Santa Body v25 (Autodesk Fusion 360 design; units mm, degrees)
Autodesk Fusion 360 part; units mm, degrees
sketch "Sketch1" plane through (0, 0, 0) normal (0, 1, 0) x (1, 0, 0)
  line L0 (55.0356, 82.2427) -> (55.0356, 73.8917)
  spline S0 degree 3 poles (10.235, 105.7553) (11.1266, 105.7379) (11.5873, 104.8858) (11.5794, 104.5647) knots 0 0 0 0 1 1 1 1
  spline S1 degree 3 poles (55.0356, 82.2427) (55.0356, 83.8658) (53.7211, 85.1817) (52.0987, 85.1817) knots 0 0 0 0 1 1 1 1
  spline S2 degree 3 poles (38.6811, 112.0285) (38.6811, 112.3322) (38.9274, 112.5785) (39.2311, 112.5785) knots 0 0 0 0 1 1 1 1
  spline S3 degree 3 poles (22.9591, 112.0969) (22.9591, 112.4007) (23.2054, 112.6469) (23.5091, 112.6469) knots 0 0 0 0 1 1 1 1
  spline S4 degree 3 poles (18.5903, 27.8928) (18.5903, 29.3352) (19.3689, 30.5045) (21.0261, 30.5045) knots 0 0 0 0 1 1 1 1
  spline S5 degree 3 poles (26.8266, 106.1753) (27.7269, 106.1753) (28.4266, 105.5866) (28.4565, 104.8612) knots 0 0 0 0 1 1 1 1
  spline S6 degree 3 poles (45.7572, 114.0087) (45.481, 114.0087) (45.2572, 114.2326) (45.2572, 114.5087) knots 0 0 0 0 1 1 1 1
  spline S7 degree 3 poles (10.235, 114.5284) (8.6125, 114.5284) (7.297, 113.2125) (7.297, 111.5894) knots 0 0 0 0 1 1 1 1
  line L1 (39.2311, 111.5335) -> (39.2311, 112.5235)
  line L2 (21.4641, 112.0969) -> (20.4741, 112.0969)
  spline S8 degree 3 poles (14.5168, 97.0703) (12.8944, 97.0703) (11.5794, 95.7544) (11.5794, 94.1313) knots 0 0 0 0 1 1 1 1
  spline S9 degree 3 poles (52.0987, 42.6031) (51.0209, 42.5992) (50.737, 43.4395) (50.7482, 43.786) knots 0 0 0 0 1 1 1 1
  line L3 (33.1192, 46.765) -> (30.3886, 46.7831)
  line L4 (29.7315, 25.7971) -> (29.7315, 27.8928)
  line L5 (45.7572, 114.9587) -> (45.7572, 114.0587)
  spline S10 degree 3 poles (11.5794, 43.7193) (11.5828, 43.2312) (11.1144, 42.5873) (10.235, 42.6031) knots 0 0 0 0 1 1 1 1
  spline S11 degree 3 poles (14.8657, 84.9034) (14.1399, 84.9034) (13.362, 85.633) (13.362, 86.5333) knots 0 0 0 0 1 1 1 1
  line L6 (47.8108, 120.2947) -> (14.5168, 120.2947)
  line L7 (39.2311, 112.5235) -> (39.2311, 111.5335)
  line L8 (13.362, 87.7791) -> (13.362, 86.5333)
  line L9 (11.5794, 117.3562) -> (11.5794, 115.708)
  spline S12 degree 3 poles (47.8108, 100.5358) (49.4323, 100.5897) (50.7482, 101.8518) (50.7482, 103.4749) knots 0 0 0 0 1 1 1 1
  spline S13 degree 3 poles (20.5642, 104.8612) (20.5642, 105.587) (21.2944, 106.1753) (22.1947, 106.1753) knots 0 0 0 0 1 1 1 1
  line L10 (27.1821, 15.6906) -> (27.1821, 15.8565)
  spline S14 degree 3 poles (39.2311, 112.5785) (39.5349, 112.5785) (39.7811, 112.3322) (39.7811, 112.0285) knots 0 0 0 0 1 1 1 1
  spline S15 degree 3 poles (21.5191, 112.0969) (21.5191, 111.7932) (21.2729, 111.5469) (20.9691, 111.5469) knots 0 0 0 0 1 1 1 1
  line L11 (46.2072, 114.5087) -> (45.7572, 114.5087)
  spline S16 degree 3 poles (34.2572, 114.5087) (34.2572, 114.7849) (34.481, 115.0087) (34.7572, 115.0087) knots 0 0 0 0 1 1 1 1
  line L12 (34.7572, 114.0587) -> (34.7572, 114.9587)
  line L13 (7.297, 73.8917) -> (7.297, 82.2427)
  line L14 (21.0261, 30.5045) -> (27.2951, 30.5045)
  line L15 (34.7572, 114.5087) -> (34.3072, 114.5087)
  line L16 (45.3072, 114.5087) -> (46.2072, 114.5087)
  line L17 (47.8108, 97.0703) -> (31.1635, 97.0703)
  line L18 (11.5794, 94.1313) -> (11.5794, 86.3718)
  line L19 (11.5794, 104.5647) -> (11.5794, 103.4749)
  line L20 (33.0945, 89.2552) -> (33.1192, 46.765)
  line L21 (45.7572, 114.5087) -> (45.3072, 114.5087)
  spline S17 degree 3 poles (34.7572, 114.9587) (35.0057, 114.9587) (35.2072, 114.7573) (35.2072, 114.5087) knots 0 0 0 0 1 1 1 1
  spline S18 degree 3 poles (29.7315, 25.7971) (29.7315, 24.3547) (28.9523, 23.1855) (27.2951, 23.1855) knots 0 0 0 0 1 1 1 1
  spline S19 degree 3 poles (35.3373, 12.025) (36.9598, 12.025) (38.2753, 13.3404) (38.2753, 14.9635) knots 0 0 0 0 1 1 1 1
  line L22 (30.3965, 89.2751) -> (33.0945, 89.2552)
  spline S20 degree 3 poles (20.9691, 111.5469) (20.6654, 111.5469) (20.4191, 111.7932) (20.4191, 112.0969) knots 0 0 0 0 1 1 1 1
  spline S21 degree 3 poles (50.7482, 104.5729) (50.749, 105.0607) (51.0594, 105.7079) (52.0987, 105.7553) knots 0 0 0 0 1 1 1 1
  spline S22 degree 3 poles (39.2311, 111.4785) (38.9274, 111.4785) (38.6811, 111.7247) (38.6811, 112.0285) knots 0 0 0 0 1 1 1 1
  line L23 (24.0041, 112.0969) -> (23.0141, 112.0969)
  spline S23 degree 3 poles (55.0356, 111.5894) (55.0356, 113.2125) (53.7211, 114.5284) (52.0987, 114.5284) knots 0 0 0 0 1 1 1 1
  line L24 (50.7482, 69.7345) -> (50.7482, 43.786)
  spline S24 degree 3 poles (50.7482, 69.7345) (50.7292, 70.4446) (51.1934, 70.9205) (52.0987, 70.9521) knots 0 0 0 0 1 1 1 1
  spline S25 degree 3 poles (52.0987, 105.7553) (53.7211, 105.7553) (55.0356, 107.0707) (55.0356, 108.6938) knots 0 0 0 0 1 1 1 1
  line L25 (11.5794, 86.3718) -> (11.5794, 94.1313)
  line L26 (34.3072, 114.5087) -> (35.2072, 114.5087)
  spline S26 degree 3 poles (45.2572, 114.5087) (45.2572, 114.7849) (45.481, 115.0087) (45.7572, 115.0087) knots 0 0 0 0 1 1 1 1
  spline S27 degree 3 poles (15.2169, 89.409) (15.9427, 89.409) (16.7206, 88.6794) (16.7206, 87.7791) knots 0 0 0 0 1 1 1 1
  line L27 (11.5794, 43.7193) -> (11.5794, 69.7582)
  spline S28 degree 3 poles (52.0987, 70.9521) (53.7202, 71.006) (55.0356, 72.2686) (55.0356, 73.8917) knots 0 0 0 0 1 1 1 1
  line L28 (13.362, 86.5333) -> (13.362, 87.7791)
  line L29 (55.0356, 111.5894) -> (55.0356, 108.6938)
  spline S29 degree 3 poles (7.297, 31.3131) (7.297, 29.69) (8.6125, 28.374) (10.235, 28.374) knots 0 0 0 0 1 1 1 1
  line L30 (0.1406, 0.1406) -> (0.1406, 121.8594)
  line L31 (14.8657, 89.409) -> (15.2169, 89.409)
  spline S30 degree 3 poles (41.7711, 112.5785) (42.0749, 112.5785) (42.3211, 112.3322) (42.3211, 112.0285) knots 0 0 0 0 1 1 1 1
  line L32 (14.5168, 16.4854) -> (22.8385, 16.4854)
  line L33 (18.5903, 27.8928) -> (18.5903, 25.7971)
  line L34 (39.2311, 112.0285) -> (39.7261, 112.0285)
  line L35 (18.5903, 25.7971) -> (18.5903, 27.8928)
  spline S31 degree 3 poles (28.4565, 104.6953) (28.4565, 103.9695) (27.7269, 103.3812) (26.8266, 103.3812) knots 0 0 0 0 1 1 1 1
  line L36 (14.8657, 84.9034) -> (15.2169, 84.9034)
  spline S32 degree 3 poles (41.7711, 111.4785) (41.4674, 111.4785) (41.2211, 111.7247) (41.2211, 112.0285) knots 0 0 0 0 1 1 1 1
  spline S33 degree 3 poles (50.7482, 94.1313) (50.7482, 95.7544) (49.4332, 97.0703) (47.8108, 97.0703) knots 0 0 0 0 1 1 1 1
  spline S34 degree 3 poles (16.7206, 86.5333) (16.7206, 85.633) (15.9423, 84.9332) (15.2169, 84.9034) knots 0 0 0 0 1 1 1 1
  line L37 (30.3886, 46.7831) -> (30.3965, 89.2751)
  line L38 (41.2761, 112.0285) -> (41.7711, 112.0285)
  spline S35 degree 3 poles (35.0744, 15.6906) (35.0744, 14.9648) (34.3442, 14.3765) (33.4439, 14.3765) knots 0 0 0 0 1 1 1 1
  spline S36 degree 3 poles (39.2311, 111.5335) (38.9578, 111.5335) (38.7361, 111.7551) (38.7361, 112.0285) knots 0 0 0 0 1 1 1 1
  spline S37 degree 3 poles (34.7572, 115.0087) (35.0333, 115.0087) (35.2572, 114.7849) (35.2572, 114.5087) knots 0 0 0 0 1 1 1 1
  line L39 (28.4565, 104.6953) -> (28.4565, 104.8612)
  line L40 (33.4439, 14.3765) -> (28.812, 14.3765)
  spline S38 degree 3 poles (10.235, 70.9521) (11.1129, 70.9036) (11.6031, 70.3892) (11.5794, 69.7582) knots 0 0 0 0 1 1 1 1
  line L41 (28.812, 17.1706) -> (33.4439, 17.1706)
  line L42 (11.5794, 115.708) -> (11.5794, 117.3562)
  line L43 (20.9691, 111.6019) -> (20.9691, 112.5919)
  line L44 (0.1406, 121.8594) -> (61.8594, 121.8594)
  line L45 (7.297, 31.3131) -> (7.297, 39.6646)
  line L46 (42.2661, 112.0285) -> (41.2761, 112.0285)
  line L47 (7.297, 39.6646) -> (7.297, 31.3131)
  line L48 (11.5794, 27.2452) -> (11.5794, 19.4245)
  line L49 (35.0744, 15.6906) -> (35.0744, 15.8565)
  spline S39 degree 3 poles (24.0041, 112.0969) (24.0041, 112.3703) (23.7825, 112.5919) (23.5091, 112.5919) knots 0 0 0 0 1 1 1 1
  line L50 (27.2951, 30.5045) -> (21.0261, 30.5045)
  line L51 (27.1821, 15.8565) -> (27.1821, 15.6906)
  spline S40 degree 3 poles (41.2211, 112.0285) (41.2211, 112.3322) (41.4674, 112.5785) (41.7711, 112.5785) knots 0 0 0 0 1 1 1 1
  line L52 (28.4565, 104.8612) -> (28.4565, 104.6953)
  spline S41 degree 3 poles (23.5091, 111.6019) (23.2357, 111.6019) (23.0141, 111.8236) (23.0141, 112.0969) knots 0 0 0 0 1 1 1 1
  line L53 (7.297, 111.5894) -> (7.297, 108.6938)
  spline S42 degree 3 poles (46.2572, 114.5087) (46.2572, 114.2326) (46.0333, 114.0087) (45.7572, 114.0087) knots 0 0 0 0 1 1 1 1
  spline S43 degree 3 poles (47.8108, 16.4854) (49.4323, 16.5393) (50.7482, 17.8014) (50.7482, 19.4245) knots 0 0 0 0 1 1 1 1
  spline S44 degree 3 poles (20.9691, 111.6019) (20.6957, 111.6019) (20.4741, 111.8236) (20.4741, 112.0969) knots 0 0 0 0 1 1 1 1
  spline S45 degree 3 poles (42.2661, 112.0285) (42.2661, 112.3019) (42.0445, 112.5235) (41.7711, 112.5235) knots 0 0 0 0 1 1 1 1
  line L54 (35.0744, 15.8565) -> (35.0744, 15.6906)
  line L55 (50.7482, 19.4245) -> (50.7482, 27.1735)
  line L56 (35.2072, 114.5087) -> (34.7572, 114.5087)
  spline S46 degree 3 poles (24.0591, 112.0969) (24.0591, 111.7932) (23.8129, 111.5469) (23.5091, 111.5469) knots 0 0 0 0 1 1 1 1
  line L57 (22.1947, 103.3812) -> (26.8266, 103.3812)
  line L58 (22.8385, 16.4854) -> (14.5168, 16.4854)
  spline S47 degree 3 poles (45.7572, 114.9587) (46.0057, 114.9587) (46.2072, 114.7573) (46.2072, 114.5087) knots 0 0 0 0 1 1 1 1
  line L59 (26.9903, 12.025) -> (35.3373, 12.025)
  line L60 (27.2951, 23.1855) -> (21.0261, 23.1855)
  line L61 (50.7482, 117.3562) -> (50.7482, 115.7102)
  spline S48 degree 3 poles (50.7482, 27.1735) (50.7463, 28.0057) (51.624, 28.3964) (52.0987, 28.374) knots 0 0 0 0 1 1 1 1
  spline S49 degree 3 poles (27.2951, 30.5045) (28.9523, 30.5045) (29.7315, 29.3352) (29.7315, 27.8928) knots 0 0 0 0 1 1 1 1
  line L62 (50.7482, 43.786) -> (50.7482, 69.7345)
  line L63 (21.0261, 23.1855) -> (27.2951, 23.1855)
  line L64 (50.7482, 103.4749) -> (50.7482, 104.5729)
  spline S50 degree 3 poles (27.1821, 15.8565) (27.1821, 16.5823) (27.9117, 17.1706) (28.812, 17.1706) knots 0 0 0 0 1 1 1 1
  spline S51 degree 3 poles (11.5794, 86.3718) (11.585, 85.8428) (11.1354, 85.1501) (10.235, 85.1817) knots 0 0 0 0 1 1 1 1
  spline S52 degree 3 poles (11.5794, 103.4749) (11.5794, 101.8518) (12.8944, 100.5358) (14.5168, 100.5358) knots 0 0 0 0 1 1 1 1
  line L65 (41.7711, 112.5235) -> (41.7711, 111.5335)
  spline S53 degree 3 poles (38.2753, 14.9635) (38.2769, 16.2773) (39.0062, 16.4966) (39.4957, 16.4854) knots 0 0 0 0 1 1 1 1
  line L66 (20.4741, 112.0969) -> (20.9691, 112.0969)
  spline S54 degree 3 poles (52.0987, 85.1817) (51.0422, 85.1715) (50.7324, 85.8189) (50.7482, 86.3525) knots 0 0 0 0 1 1 1 1
  spline S55 degree 3 poles (50.7482, 117.3562) (50.7482, 118.9793) (49.4332, 120.2947) (47.8108, 120.2947) knots 0 0 0 0 1 1 1 1
  line L67 (23.5091, 111.6019) -> (23.5091, 112.5919)
  line L68 (20.5642, 104.8612) -> (20.5642, 104.6953)
  spline S56 degree 3 poles (10.235, 85.1817) (8.6125, 85.1817) (7.297, 83.8658) (7.297, 82.2427) knots 0 0 0 0 1 1 1 1
  line L69 (47.8108, 100.5358) -> (14.5168, 100.5358)
  spline S57 degree 3 poles (20.9691, 112.6469) (21.2729, 112.6469) (21.5191, 112.4007) (21.5191, 112.0969) knots 0 0 0 0 1 1 1 1
  line L70 (45.7572, 114.0587) -> (45.7572, 114.9587)
  line L71 (11.5794, 103.4749) -> (11.5794, 104.5647)
  line L72 (28.812, 14.3765) -> (33.4439, 14.3765)
  spline S58 degree 3 poles (28.812, 14.3765) (27.9117, 14.3765) (27.212, 14.9652) (27.1821, 15.6906) knots 0 0 0 0 1 1 1 1
  spline S59 degree 3 poles (22.8385, 16.4854) (23.3022, 16.5043) (24.0076, 16.1123) (24.0523, 14.9635) knots 0 0 0 0 1 1 1 1
  spline S60 degree 3 poles (13.362, 87.7791) (13.362, 88.6794) (14.1399, 89.409) (14.8657, 89.409) knots 0 0 0 0 1 1 1 1
  line L73 (14.5168, 120.2947) -> (47.8108, 120.2947)
  spline S61 degree 3 poles (14.5168, 120.2947) (12.8944, 120.2947) (11.5794, 118.9793) (11.5794, 117.3562) knots 0 0 0 0 1 1 1 1
  line L74 (50.7482, 86.3525) -> (50.7482, 94.1313)
  spline S62 degree 3 poles (55.0356, 39.6646) (55.0356, 41.2877) (53.7211, 42.6031) (52.0987, 42.6031) knots 0 0 0 0 1 1 1 1
  line L75 (39.7261, 112.0285) -> (38.7361, 112.0285)
  line L76 (7.297, 108.6938) -> (7.297, 111.5894)
  line L77 (23.5091, 112.5919) -> (23.5091, 111.6019)
  spline S63 degree 3 poles (23.5091, 111.5469) (23.2054, 111.5469) (22.9591, 111.7932) (22.9591, 112.0969) knots 0 0 0 0 1 1 1 1
  line L78 (16.7206, 86.5333) -> (16.7206, 87.7791)
  spline S64 degree 3 poles (24.0523, 14.9635) (24.1061, 13.3413) (25.3678, 12.025) (26.9903, 12.025) knots 0 0 0 0 1 1 1 1
  line L79 (61.8594, 0.1406) -> (0.1406, 0.1406)
  line L80 (31.1635, 97.0703) -> (14.5168, 97.0703)
  line L81 (39.4957, 16.4854) -> (47.8108, 16.4854)
  spline S65 degree 3 poles (10.235, 28.374) (10.7285, 28.3793) (11.6383, 28.108) (11.5794, 27.2452) knots 0 0 0 0 1 1 1 1
  line L82 (47.8108, 16.4854) -> (39.4957, 16.4854)
  line L83 (41.7711, 111.5335) -> (41.7711, 112.5235)
  line L84 (55.0356, 108.6938) -> (55.0356, 111.5894)
  line L85 (41.7711, 112.0285) -> (42.2661, 112.0285)
  spline S66 degree 3 poles (45.3072, 114.5087) (45.3072, 114.2602) (45.5086, 114.0587) (45.7572, 114.0587) knots 0 0 0 0 1 1 1 1
  line L86 (50.7482, 104.5729) -> (50.7482, 103.4749)
  spline S67 degree 3 poles (52.0987, 28.374) (53.7202, 28.4279) (55.0356, 29.69) (55.0356, 31.3131) knots 0 0 0 0 1 1 1 1
  line L87 (29.7315, 27.8928) -> (29.7315, 25.7971)
  line L88 (15.2169, 84.9034) -> (14.8657, 84.9034)
  spline S68 degree 3 poles (35.2572, 114.5087) (35.2572, 114.2326) (35.0333, 114.0087) (34.7572, 114.0087) knots 0 0 0 0 1 1 1 1
  line L89 (33.4439, 17.1706) -> (28.812, 17.1706)
  spline S69 degree 3 poles (34.3072, 114.5087) (34.3072, 114.2602) (34.5086, 114.0587) (34.7572, 114.0587) knots 0 0 0 0 1 1 1 1
  line L90 (50.7482, 27.1735) -> (50.7482, 19.4245)
  line L91 (11.5794, 69.7582) -> (11.5794, 43.7193)
  line L92 (50.7482, 115.7102) -> (50.7482, 117.3562)
  line L93 (34.7572, 114.9587) -> (34.7572, 114.0587)
  line L94 (16.7206, 87.7791) -> (16.7206, 86.5333)
  spline S70 degree 3 poles (7.297, 108.6938) (7.3508, 107.0716) (8.6125, 105.7553) (10.235, 105.7553) knots 0 0 0 0 1 1 1 1
  line L95 (50.7482, 94.1313) -> (50.7482, 86.3525)
  spline S71 degree 3 poles (20.4191, 112.0969) (20.4191, 112.4007) (20.6654, 112.6469) (20.9691, 112.6469) knots 0 0 0 0 1 1 1 1
  spline S72 degree 3 poles (21.4641, 112.0969) (21.4641, 112.3703) (21.2425, 112.5919) (20.9691, 112.5919) knots 0 0 0 0 1 1 1 1
  line L96 (55.0356, 73.8917) -> (55.0356, 82.2427)
  line L97 (61.8594, 121.8594) -> (61.8594, 0.1406)
  spline S73 degree 3 poles (21.0261, 23.1855) (19.3689, 23.1855) (18.6453, 24.3555) (18.5903, 25.7971) knots 0 0 0 0 1 1 1 1
  line L98 (20.5642, 104.6953) -> (20.5642, 104.8612)
  line L99 (7.297, 82.2427) -> (7.297, 73.8917)
  spline S74 degree 3 poles (42.3211, 112.0285) (42.3211, 111.7247) (42.0749, 111.4785) (41.7711, 111.4785) knots 0 0 0 0 1 1 1 1
  line L100 (22.1947, 106.1753) -> (26.8266, 106.1753)
  line L101 (55.0356, 39.6646) -> (55.0356, 31.3131)
  line L102 (11.5794, 19.4245) -> (11.5794, 27.2452)
  line L103 (26.8266, 103.3812) -> (22.1947, 103.3812)
  line L104 (20.9691, 112.0969) -> (21.4641, 112.0969)
  spline S75 degree 3 poles (34.7572, 114.0087) (34.481, 114.0087) (34.2572, 114.2326) (34.2572, 114.5087) knots 0 0 0 0 1 1 1 1
  spline S76 degree 3 poles (7.297, 73.8917) (7.297, 72.2686) (8.6125, 70.9521) (10.235, 70.9521) knots 0 0 0 0 1 1 1 1
  spline S77 degree 3 poles (11.5794, 19.4245) (11.5794, 17.8014) (12.8944, 16.4854) (14.5168, 16.4854) knots 0 0 0 0 1 1 1 1
  line L105 (14.5168, 97.0703) -> (47.8108, 97.0703)
  line L106 (23.0141, 112.0969) -> (23.5091, 112.0969)
  spline S78 degree 3 poles (33.4439, 17.1706) (34.3442, 17.1706) (35.0744, 16.5823) (35.0744, 15.8565) knots 0 0 0 0 1 1 1 1
  line L107 (26.8266, 106.1753) -> (22.1947, 106.1753)
  spline S79 degree 3 poles (52.0987, 114.5284) (51.2509, 114.5136) (50.7594, 115.2803) (50.7482, 115.7102) knots 0 0 0 0 1 1 1 1
  line L108 (15.2169, 89.409) -> (14.8657, 89.409)
  line L109 (38.7361, 112.0285) -> (39.2311, 112.0285)
  spline S80 degree 3 poles (22.1947, 103.3812) (21.2944, 103.3812) (20.5642, 103.9695) (20.5642, 104.6953) knots 0 0 0 0 1 1 1 1
  spline S81 degree 3 poles (39.7261, 112.0285) (39.7261, 112.3019) (39.5045, 112.5235) (39.2311, 112.5235) knots 0 0 0 0 1 1 1 1
  spline S82 degree 3 poles (39.7811, 112.0285) (39.7811, 111.7247) (39.5349, 111.4785) (39.2311, 111.4785) knots 0 0 0 0 1 1 1 1
  line L110 (20.9691, 112.5919) -> (20.9691, 111.6019)
  spline S83 degree 3 poles (45.7572, 115.0087) (46.0333, 115.0087) (46.2572, 114.7849) (46.2572, 114.5087) knots 0 0 0 0 1 1 1 1
  line L111 (14.5168, 100.5358) -> (47.8108, 100.5358)
  line L112 (35.3373, 12.025) -> (26.9903, 12.025)
  spline S84 degree 3 poles (10.235, 42.6031) (8.6125, 42.6031) (7.297, 41.2877) (7.297, 39.6646) knots 0 0 0 0 1 1 1 1
  spline S85 degree 3 poles (23.5091, 112.6469) (23.8129, 112.6469) (24.0591, 112.4007) (24.0591, 112.0969) knots 0 0 0 0 1 1 1 1
  line L113 (23.5091, 112.0969) -> (24.0041, 112.0969)
  spline S86 degree 3 poles (41.7711, 111.5335) (41.4978, 111.5335) (41.2761, 111.7551) (41.2761, 112.0285) knots 0 0 0 0 1 1 1 1
  line L114 (55.0356, 31.3131) -> (55.0356, 39.6646)
  spline S87 degree 3 poles (11.5794, 115.708) (11.6016, 114.9323) (11.1123, 114.6075) (10.235, 114.5284) knots 0 0 0 0 1 1 1 1
  line L115 (21.8777, 89.1799) -> (42.6944, 87.5532)
  spline S88 degree 3 poles (-9.3705, 49.5169) (-8.0356, 47.9653) (-5.5333, 47.611) (-2.9224, 48.6041) knots 0 0 0 0 1 1 1 1
  spline S89 degree 3 poles (65.2052, 60.389) (65.4072, 63.3249) (65.518, 66.8134) (65.4808, 71.2232) knots 0 0 0 0 1 1 1 1
  line L116 (22.004, 31.0011) -> (22.004, 29.5592)
  spline S90 degree 3 poles (-6.9578, 58.456) (-10.217, 55.7643) (-11.2972, 51.7622) (-9.3705, 49.5169) knots 0 0 0 0 1 1 1 1
  line L117 (38.7177, 31.1546) -> (13.9635, 30.9272)
  line L118 (42.6944, 87.5532) -> (37.9564, 89.1831)
  spline S91 degree 3 poles (-2.9224, 48.6041) (-2.569, 47.0681) (-2.2507, 45.7402) (-2.0454, 44.9143) knots 0 0 0 0 1 1 1 1
  line L119 (33.5618, 31.1072) -> (38.7177, 31.1546)
  spline S92 degree 3 poles (-2.4169, 45.7632) (-3.8924, 34.8262) (4.3175, 31.5493) (13.9635, 30.9272) knots 0 0 0 0 1 1 1 1
  spline S93 degree 3 poles (-5.8862, 68.9158) (-6.0232, 66.9046) (-5.7737, 64.1092) (-5.3427, 61.1145) knots 0 0 0 0 1 1 1 1
  spline S94 degree 3 poles (63.847, 49.7627) (65.5565, 49.6449) (67.0162, 50.1665) (67.9193, 51.2179) knots 0 0 0 0 1 1 1 1
  spline S95 degree 3 poles (-6.3178, 59.0425) (-6.3039, 59.0194) (-6.289, 58.9966) (-6.2732, 58.9741) knots 0 0 0 0 1 1 1 1
  spline S96 degree 3 poles (38.7177, 31.1546) (42.5891, 31.2922) (65.3304, 34.0027) (63.2742, 46.2404) knots 0 0 0 0 1 1 1 1
  spline S97 degree 3 poles (63.2274, 46.2233) (63.4316, 47.4338) (63.6405, 48.5943) (63.847, 49.7627) knots 0 0 0 0 1 1 1 1
  line L120 (21.8777, 89.1799) -> (15.6125, 86.6019)
  line L121 (33.5618, 29.5592) -> (33.5618, 31.1072)
  spline S98 degree 3 poles (65.5067, 60.157) (65.4075, 60.2361) (65.307, 60.3135) (65.2052, 60.389) knots 0 0 0 0 1 1 1 1
  spline S99 degree 3 poles (-6.2732, 58.9741) (-6.5078, 58.8107) (-6.7363, 58.6377) (-6.9578, 58.456) knots 0 0 0 0 1 1 1 1
  spline S100 degree 3 poles (-2.0454, 44.9143) (-2.1777, 45.1904) (-2.3031, 45.4723) (-2.4169, 45.7632) knots 0 0 0 0 1 1 1 1
  line L122 (22.004, 29.5592) -> (33.5618, 29.5592)
  spline S101 degree 3 poles (67.9193, 51.2179) (69.846, 53.4631) (68.7658, 57.4652) (65.5067, 60.157) knots 0 0 0 0 1 1 1 1
  spline S102 degree 3 poles (63.2742, 46.2404) (63.2603, 46.2368) (63.2422, 46.2281) (63.2274, 46.2233) knots 0 0 0 0 1 1 1 1
  line L123 (37.9564, 89.1831) -> (21.8777, 89.1799)
  line L124 (15.6125, 86.6019) -> (21.8777, 89.1799)
  spline S103 degree 3 poles (15.6125, 86.6019) (6.6175, 84.838) (-3.4606, 80.3637) (-5.8862, 68.9158) knots 0 0 0 0 1 1 1 1
  spline S104 degree 3 poles (-5.3427, 61.1145) (-6.3033, 60.4856) (-6.6808, 59.6832) (-6.3178, 59.0425) knots 0 0 0 0 1 1 1 1
  line L125 (13.9635, 30.9272) -> (22.004, 31.0011)
  spline S105 degree 3 poles (65.4808, 71.2232) (64.7586, 79.2544) (53.1536, 87.8198) (42.6944, 87.5532) knots 0 0 0 0 1 1 1 1
  line L126 (21.7497, 68.031) -> (21.7413, 110.7625) construction
  line L127 (41.7582, 25) -> (41.7455, 89.4956) construction
  line L128 (31.7539, 46.774) -> (31.7455, 89.2651) construction
  line L129 (20.2955, 25) -> (23.1955, 25)
  line L130 (23.1955, 25) -> (23.1955, 89.3968)
  line L131 (23.1955, 89.3968) -> (20.2955, 89.3968)
  line L132 (20.2955, 89.3968) -> (20.2955, 25)
  line L133 (44.2106, 89.3968) -> (17, 89.3968) construction
  line L134 (44.7035, 46.7674) -> (16.8671, 46.7512) construction
  line L135 (40.3082, 89.3968) -> (43.2082, 89.3968)
  line L136 (43.2082, 89.3968) -> (43.2082, 25)
  line L137 (43.2082, 25) -> (40.3082, 25)
  line L138 (40.3082, 25) -> (40.3082, 89.3968)
  line L139 (7, 25) -> (55, 25) construction
  circle A0 centre (31.7539, 46.774) radius 2
  dimension "d11" = 10
  dimension "d12" = 10
  dimension "d17" = 2.9
  dimension "d18" = 2.9
  dimension "d23" = 4
  constraint midpoint L3
  constraint midpoint L22
  constraint perpendicular L123 L128
  constraint vertical L130
  constraint horizontal L131
  constraint vertical L132
  constraint perpendicular L132 L133
  constraint collinear L131 L133
  constraint midpoint L126 L131
  constraint perpendicular L20 L134
  constraint horizontal L135
  constraint vertical L136
  constraint vertical L138
  constraint coincident L133
  constraint midpoint origin L137
  constraint parallel L60 L139
  constraint collinear L129 L139
  constraint collinear L137 L139
  measures "d11" distance of L126 L128
  measures "d12" distance of L127 L128
  measures "d23" diameter of A0
extrude "Extrude1" add sketch "Sketch1" along normal blind 3 contours L0 S1 S9 L24 S24 S28 L62 S54 S62 L96 L97 L101 L114 S96 S105 | L0 S1 S9 L24 S24 S28 L62 S54 S62 L96 L101 L114 S96 S105 L136 | L97 S89 S94 S96 S97 S98 S101 S102 S105 | L115 S96 S105 L136 L138 | L20 L37 L115 L117 L119 S96 L130 L138 A0 | S10 L13 L27 L30 S38 L45 L47 S56 L91 L99 S76 S84 S92 S103 | L30 S88 S90 S91 S92 S93 S95 S99 S100 S103 S104 | L20 L37 L115 A0 | S10 S11 L13 L27 L36 S34 S38 L45 L47 S51 S56 L78 L88 L91 L94 L99 S76 S84 L117 S92 L120 L124 S103 L125 L132 | L3 L20 L37 A0 | L3 L20 L37 A0 | L115 L117 L120 L124 L125 L130 L132 | S11 L36 S34 L78 L88 L94 L120 L124 S103
extrude "Extrude2" cut sketch "Sketch1" along normal blind 2.1 contours L115 S96 S105 L136 L138 | L118 S105 L135 L136 L138 | L115 L118 L138 | S96 L136 L137 L138 | L115 L117 L120 L124 L125 L130 L132 | L115 L123 L130 | L14 L50 L116 L117 L130 | L120 L123 L124 L130 L131 L132 | S4 L14 L50 L116 L117 L125 L132 | L14 L50 L116 L122 L130 | S4 L14 L50 L116 L122 L129 L130 L132
extrude "Extrude5" cut sketch "Sketch1" along normal through all contours L3 L20 L37 A0 | L3 L20 L37 A0
extrude "Extrude4" [suppressed]
extrude "Extrude3" [suppressed]
